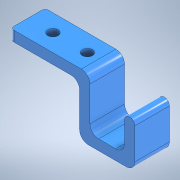
# Autodesk Inventor part: Cable_Guide_Holder
Saved by Autodesk Inventor 2022 (Build 260153000, 153)
## iProperties
Created: 2021-08-21
Part Number: Cable_Guide_Holder
Material: Generic
Document SubType Name: Modeling
Designer: Jorian Bruslind
Density: 1 g/cm^3
Appearance: Cyan
Author: Jorian Bruslind
Autodesk Inventor part; units mm, degrees
ref_plane "YZ Plane" through (0, 0, 0) normal (1, 0, 0) x (0, 1, 0)
ref_plane "XZ Plane" through (0, 0, 0) normal (0, 1, 0) x (-1, 0, 0)
ref_plane "XY Plane" through (0, 0, 0) normal (0, 0, 1) x (1, 0, 0)
sketch "Sketch1" plane through (0, 0, 0) normal (0, 1, 0) x (-1, 0, 0)
  line L0 (0, 0) -> (40, 0)
  line L1 (40, 0) -> (40, -20)
  line L2 (40, -20) -> (0, -20)
  line L3 (0, -20) -> (0, 0)
  dimension "d0" = 40
  dimension "d1" = 20
  constraints: 8 end point, 2 parallel, 1 horizontal, 1 perpendicular
  measures "d0" distance of L1.end L2.end
  measures "d1" distance of L0.end L1.end
extrude "Extrusion1" add sketch "Sketch1" along normal blind 6
sketch "Sketch2" plane through (0, 6, 0) normal (0, 1, 0) x (1, 0, 0)
  line L0 (0, 0) -> (6, 0)
  line L1 (6, 0) -> (6, 20)
  line L2 (6, 20) -> (0, 20)
  line L3 (0, 20) -> (0, 0)
  dimension "d4" = 6
  dimension "d5" = 20
  constraints: 8 end point, 2 parallel, 1 horizontal, 1 perpendicular
  measures "d4" distance of L2.end L1.end
  measures "d5" distance of L1.end L0.end
extrude "Extrusion2" add sketch "Sketch2" against normal blind 30
fillet "Fillet1" radius 5 1 edges at (0, 0, -10)
fillet "Fillet4" radius 5 1 edges at (6, 6, -10)
sketch "Sketch5" plane through (0, 0, 0) normal (0, -1, 0) x (1, 0, 0)
  circle A0 centre (-5.5, -10) radius 3
  line L0 (-40, -20) -> (-40, 0) projected
  line L1 (-5, -20) -> (-40, -20) projected
  line L2 (6, -20) -> (6, 0) projected
  circle A1 centre (-25.5, -10) radius 3
  line L3 (-40, 0) -> (-5, 0) projected
  point P0 (0, 0)
  dimension "d18" = 6
  dimension "d20" = 10
  dimension "d47" = 11.5
  dimension "d48" = 6
  dimension "d49" = 20
  dimension "d50" = 10
  constraints: 2 centre point
  measures "d18" diameter of A0
  measures "d20" distance from line of L1 A0.centre
  measures "d47" distance from line of L2 A0.centre
  measures "d48" diameter of A1
  measures "d49" distance of A0.centre A1.centre
  measures "d50" distance from line of L3 A1.centre
fillet "Fillet7" radius 2 2 edges at (-40, 3, 0) (-40, 3, -20)
sketch "Sketch8" plane through (0, -24, -20) normal (-1, 0, 0) x (0, 0, 1)
  line L0 (20, 0) -> (0, 0) projected
  line L1 (0, 0) -> (20, 0)
  line L2 (20, 0) -> (20, -6)
  line L3 (20, -6) -> (0, -6)
  line L4 (0, -6) -> (0, 0)
  point P0 (20, 24)
  dimension "d35" = 6
  constraints: 8 end point, 2 parallel, 1 horizontal, 1 perpendicular
  measures "d35" distance of L1.end L2.end
extrude "Extrusion6" add sketch "Sketch8" against normal blind 32
fillet "Fillet8" radius 5 1 edges at (0, -30, -10)
fillet "Fillet9" radius 5 1 edges at (6, -24, -10)
sketch "Sketch9" plane through (32, -24, 0) normal (0, 1, 0) x (1, 0, 0)
  line L0 (0, 20) -> (0, 0) projected
  line L1 (0, 20) -> (-6, 20)
  line L2 (-6, 20) -> (-6, 0)
  line L3 (-6, 0) -> (0, 0)
  line L4 (0, 0) -> (0, 20)
  point P0 (-32, 0)
  dimension "d40" = 6
  dimension "d41" = 20
  constraints: 8 end point, 2 parallel, 1 horizontal, 1 perpendicular
  measures "d40" distance of L3.end L2.end
  measures "d41" distance of L2.end L1.end
extrude "Extrusion7" add sketch "Sketch9" along normal blind 20
fillet "Fillet10" radius 5 1 edges at (26, -24, -10)
fillet "Fillet11" radius 5 1 edges at (32, -30, -10)
fillet "Fillet12" radius 3 2 edges at (26, -4, -10) (32, -4, -10)
extrude "Extrusion8" cut sketch "Sketch5" against normal through all both and the other way through all
sketch "Sketch10" plane through (0, 0, 0) normal (0, -1, 0) x (1, 0, 0)
  circle A0 centre (-5.5, -10) radius 3 projected
  circle A1 centre (-5.5, -10) radius 5
  point P0 (0, 0)
  dimension "d53" = 10
  constraints: 1 centre point, 1 coincident
  measures "d53" diameter of A1
extrude "Extrusion9" cut sketch "Sketch10" along normal through all contours A0 | A1
body "Solid1"
